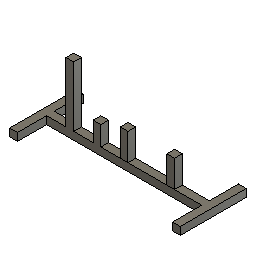
Aluminium Profile System (Autodesk Fusion 360 design; units mm, degrees)
Autodesk Fusion 360 part; units mm, degrees
sketch "Eskiz1" plane through (0, 0, 0) normal (0, 1, 0) x (1, 0, 0)
  line L0 (0, 0) -> (600, 0)
  line L1 (600, 0) -> (600, -40)
  line L2 (600, -40) -> (0, -40)
  line L3 (0, -40) -> (0, 0)
  line L4 (0, 0) -> (-100, 0)
  line L5 (-100, 0) -> (-100, -40)
  line L6 (-100, -40) -> (0, -40)
  line L7 (0, -40) -> (0, 0)
  line L8 (-100, 0) -> (-140, 0)
  line L9 (-140, 0) -> (-140, -190)
  line L10 (-140, -190) -> (-100, -190)
  line L11 (-100, -190) -> (-100, 0)
  line L12 (-100, -40) -> (-140, -40)
  line L13 (-140, -40) -> (-140, 150)
  line L14 (-140, 150) -> (-100, 150)
  line L15 (-100, 150) -> (-100, -40)
  line L16 (740, 0) -> (740, -190)
  line L17 (700, 0) -> (600, 0)
  line L18 (740, -40) -> (740, 150)
  line L19 (600, -40) -> (700, -40)
  line L20 (700, -190) -> (700, 0)
  line L21 (740, -190) -> (700, -190)
  line L22 (700, -40) -> (700, 0)
  line L23 (740, 150) -> (700, 150)
  line L24 (700, -40) -> (740, -40)
  line L25 (700, 0) -> (740, 0)
  line L26 (700, 150) -> (700, -40)
  dimension "d1" = 600
  dimension "d2" = 40
  dimension "d24" = 100
  dimension "d25" = 40
  dimension "d26" = 40
  dimension "d27" = 190
  dimension "d28" = 40
  dimension "d29" = 190
  dimension "d30" = 100
  dimension "d31" = 40
  dimension "d32" = 40
  dimension "d33" = 190
  dimension "d34" = 40
  dimension "d35" = 190
  constraint horizontal L0
  constraint vertical L1
  constraint horizontal L2
  constraint vertical L3
  constraint coincident L0.start L3.end
  constraint horizontal L4
  constraint vertical L5
  constraint horizontal L6
  constraint vertical L7
  constraint horizontal L8
  constraint vertical L9
  constraint horizontal L10
  constraint vertical L11
  constraint horizontal L12
  constraint vertical L13
  constraint horizontal L14
  constraint vertical L15
  measures "d1" distance of L0.start L0.end
  measures "d2" distance of L0.start L2.end
  measures "d24" distance of L0.start L4.end
  measures "d25" distance of L0.start L2.end
  measures "d26" distance of L4.end L8.end
  measures "d27" distance of L4.end L10.end
  measures "d28" distance of L5.end L12.end
  measures "d29" distance of L5.end L14.end
  measures "d30" distance of L1.end L19.end
  measures "d31" distance of L1.end L0.end
  measures "d32" distance of L18.start L19.end
  measures "d33" distance of L23.end L19.end
  measures "d34" distance of L16.start L17.start
  measures "d35" distance of L20.start L17.start
extrude "Ekstrüde Et1" add sketch "Eskiz1" along normal blind 40 contours L0 L1 L2 L3 L7 makes body 1
sketch "Eskiz2" plane through (0, 40, 0) normal (0, 1, 0) x (-1, 0, 0)
  line L0 (0, 40) -> (-600, 40)
  line L1 (-600, 40) -> (-600, 0)
  line L2 (-600, 0) -> (0, 0)
  line L3 (0, 0) -> (0, 40)
  line L4 (0, 0) -> (-40, 0)
  line L5 (-40, 0) -> (-40, 40)
  line L6 (-40, 40) -> (0, 40)
  line L7 (0, 40) -> (0, 0)
  line L8 (-280, 0) -> (-320, 0)
  line L9 (-320, 0) -> (-320, 40)
  line L10 (-320, 40) -> (-280, 40)
  line L11 (-280, 40) -> (-280, 0)
  line L12 (-520, 0) -> (-560, 0)
  line L13 (-560, 0) -> (-560, 40)
  line L14 (-560, 40) -> (-520, 40)
  line L15 (-520, 40) -> (-520, 0)
  line L16 (-140, 0) -> (-180, 0)
  line L17 (-180, 0) -> (-180, 40)
  line L18 (-180, 40) -> (-140, 40)
  line L19 (-140, 40) -> (-140, 0)
  dimension "d5" = 40
  dimension "d6" = 40
  dimension "d7" = 40
  dimension "d8" = 40
  dimension "d9" = 40
  dimension "d16" = 40
  dimension "d17" = 40
  dimension "d20" = 40
  dimension "d21" = 100
  dimension "d22" = 100
  dimension "d23" = 200
  constraint horizontal L4
  constraint vertical L5
  constraint horizontal L6
  constraint vertical L7
  constraint coincident L2.end L3.start
  constraint horizontal L8
  constraint vertical L9
  constraint horizontal L10
  constraint vertical L11
  constraint coincident L2 L8.start
  constraint horizontal L12
  constraint vertical L13
  constraint horizontal L14
  constraint vertical L15
  constraint coincident L2 L12.start
  constraint horizontal L16
  constraint vertical L17
  constraint horizontal L18
  constraint vertical L19
  constraint coincident L2 L16.start
  measures "d5" distance of L2.end L4.end
  measures "d6" distance of L8.start L8.end
  measures "d7" distance of L8.start L10.end
  measures "d8" distance of L12.start L12.end
  measures "d9" distance of L12.start L14.end
  measures "d16" distance of L16.start L16.end
  measures "d17" distance of L16.start L18.end
  measures "d20" distance of L2.end L0.start
  measures "d21" distance of L4.end L16.start
  measures "d22" distance of L8.start L16.end
  measures "d23" distance of L8.end L12.start
extrude "Ekstrüde Et2" add sketch "Eskiz2" along normal blind 140 separate body contours L0 L2 L8 L9 L10 L11 | L0 L2 L12 L13 L14 L15 makes body 2 at (280, 86.6667, 26.6667) makes body 3 at (520, 86.6667, 26.6667)
extrude "Ekstrüde Et3" add sketch "Eskiz2" along normal blind 310 contours L0 L2 L3 L4 L5 L6 L7 bodies 1
extrude "Ekstrüde Et4" add sketch "Eskiz1" along normal blind 40 contours L3 L4 L5 L6 L7 L11 L15 | L1 L17 L19 L20 L22 L26 | L5 L8 L9 L11 L12 L13 L15 | L8 L13 L14 L15 | L16 L18 L20 L22 L24 L25 L26 | L18 L23 L25 L26 | L9 L10 L11 L12 | L16 L20 L21 L24 bodies 1
extrude "Ekstrüde Et5" add sketch "Eskiz2" along normal blind 100 contours L0 L2 L16 L17 L18 L19 bodies 1
